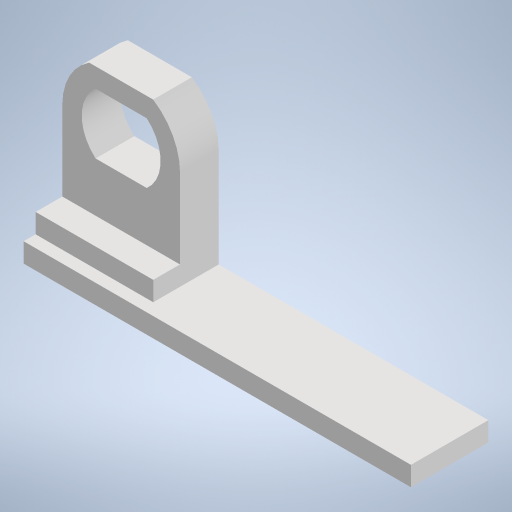
# Autodesk Inventor part: tempHolder
Saved by Autodesk Inventor 2023 (Build 270158000, 158)
## iProperties
Created: 2022-11-22
Part Number: tempHolder
Material: Generic
Document SubType Name: Modeling
Designer: shrey
Density: 1 g/cm^3
Appearance: Default
Author: shrey
Autodesk Inventor part; units mm, degrees
ref_plane "YZ Plane" through (0, 0, 0) normal (1, 0, 0) x (0, 1, 0)
ref_plane "Work Plane1" through (31.1962, 56.4165, 110.8343) normal (0, 0, 1) x (1, 0, 0)
sketch "Sketch2" plane through (31.1962, 56.4165, 110.8343) normal (0, 0, 1) x (1, 0, 0)
  line L0 (6.5, -7.5) -> (-6.5, -7.5) construction
  line L1 (-6.5, 7.5) -> (6.5, 7.5) construction
  arc A0 (6.5, -7.5) -> (6.5, 7.5) centre (-0.1144, 0) ccw construction
  arc A1 (-6.5, 7.5) -> (-6.5, -7.5) centre (0.1144, 0) ccw construction
  line L2 (6.6124, 7.8) -> (-6.6124, 7.8)
  arc A2 (-6.6124, 7.8) -> (-6.6124, -7.8) centre (0.1144, 0) ccw
  line L3 (-6.6124, -7.8) -> (6.6124, -7.8)
  arc A3 (6.6124, -7.8) -> (6.6124, 7.8) centre (-0.1144, 0) ccw
  line L4 (8.2671, 12.8) -> (-8.2671, 12.8)
  arc A4 (-8.2671, 12.8) -> (-8.2671, -12.8) centre (0.1144, 0) ccw
  line L5 (-8.2671, -12.8) -> (8.2671, -12.8)
  arc A5 (8.2671, -12.8) -> (8.2671, 12.8) centre (-0.1144, 0) ccw
  line L6 (15.1856, 0) -> (-15.1856, 0) construction
  line L7 (-15.1856, 0) -> (-15.1856, -30.6)
  line L8 (-15.1856, -30.6) -> (15.1856, -30.6)
  line L9 (15.1856, -30.6) -> (15.1856, 0)
  line L10 (15.1856, -30.6) -> (-15.1856, -30.6)
  line L11 (-15.1856, -30.6) -> (-15.1856, -25.6)
  line L12 (15.1856, -25.6) -> (15.1856, -30.6)
  line L13 (15.1856, -20.6) -> (-15.1856, -20.6)
  line L14 (-15.1856, -30.6) -> (84.8144, -30.6)
  line L15 (84.8144, -30.6) -> (84.8144, -25.6)
  line L16 (84.8144, -25.6) -> (-15.1856, -25.6)
  line L17 (-15.1856, -25.6) -> (-15.1856, -30.6)
  point P0 (-31.1962, -56.4165)
  point P1 (-15.1856, 0)
  dimension "d5" = 0.3
  dimension "d6" = 5
  dimension "d7" = 30.6
  dimension "d16" = 100
  constraints: 32 end point, 13 point on circle, 6 centre point, 5 parallel, 4 perpendicular, 3 horizontal, 3 point on line, 1 tangent, 6 other
  measures "d5" radial gap between concentric circles of A0 A3
  measures "d6" radial gap between concentric circles of A3 A5
  measures "d7" distance of L6.end L7.end
  measures "d16" distance of L16.end L15.end
extrude "Extrusion1" add sketch "Sketch2" against normal blind 10 contours A5 L5 A4 L4 | L9 L13 L7 A4 L5 A5 | L9 L16 L7 L13 | L9 L8 L7 L16
ref_plane "Work Plane2" through (-8.5806, 30.9168, 125.8343) normal (0, 0, 1) x (1, 0, 0)
extrude "Extrusion2" add sketch "Sketch2" along normal blind 10 and the other way blind 10 contours L16 L15 L14 L9 | L9 L8 L7 L16
extrude "Extrusion3" add sketch "Sketch2" along normal blind 6.9 contours L9 L16 L7 L13 | L9 L8 L7 L16
body "Solid1"
